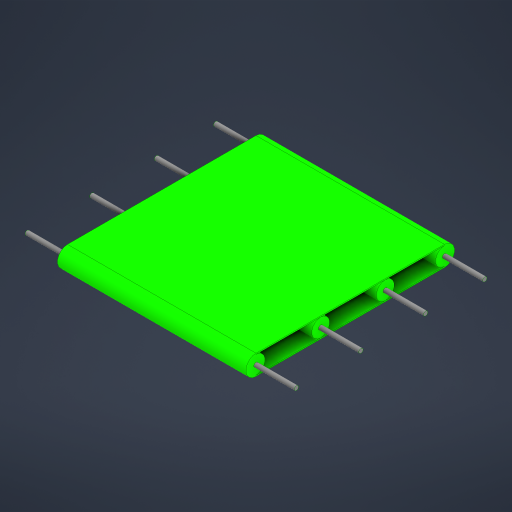
# Autodesk Inventor part: Conveyor
Saved by Autodesk Inventor 2023 (Build 270158000, 158)
## iProperties
Created: 2023-11-04
Part Number: Conveyor
Material: Generic
Document SubType Name: Modeling
Designer: Abhinav
Density: 1 g/cm^3
Appearance: Default(1)
Author: Abhinav
Autodesk Inventor part; units mm, degrees
ref_plane "YZ Plane" through (0, 0, 0) normal (1, 0, 0) x (0, 1, 0)
ref_plane "XZ Plane" through (0, 0, 0) normal (0, 1, 0) x (-1, 0, 0)
sketch "Sketch1" plane through (0, 0, 0) normal (1, 0, 0) x (0, 1, 0)
  line L0 (0, 0) -> (0, -350) construction
  line L1 (0, 0) -> (0, -350) construction
  line L2 (-16.7, 0) -> (-16.7, -350)
  line L3 (16.7, -350) -> (16.7, 0)
  arc A0 (16.7, 0) -> (-16.7, 0) centre (0, 0) ccw
  arc A1 (-16.7, -350) -> (16.7, -350) centre (0, -350) ccw
  line L4 (0, 0) -> (0, -350) construction
  line L5 (-18.7, 0) -> (-18.7, -350)
  line L6 (18.7, -350) -> (18.7, 0)
  arc A2 (18.7, 0) -> (-18.7, 0) centre (0, 0) ccw
  arc A3 (-18.7, -350) -> (18.7, -350) centre (0, -350) ccw
  circle A4 centre (0, 0) radius 16.7
  circle A5 centre (0, -350) radius 16.7
  line L7 (0, 0) -> (0, -120) construction
  line L8 (0, -120) -> (0, -240) construction
  circle A6 centre (0, -120) radius 16.7
  circle A7 centre (0, -240) radius 16.7
  point P0 (0, -175)
  point P1 (0, -175)
  point P2 (-16.7, -240)
  point P3 (-16.7, -120)
  point P4 (16.7, 0)
  point P5 (16.7, -120)
  point P6 (16.7, -240)
  point P7 (16.7, -350)
  dimension "d0" = 350
  dimension "d1" = 33.4
  dimension "d8" = 37.4
  dimension "d9" = 120
  dimension "d10" = 120
  constraints: 22 end point, 10 tangent, 8 point on circle, 6 centre point, 4 coincident, 3 equal length, 2 midpoint, 2 point on line, 2 vertical, 6 other
  measures "d0" distance of L0.start L0.end
  measures "d1" diameter of A1
  measures "d8" diameter of A3
  measures "d9" distance of L7.start L7.end
  measures "d10" distance of L7.end L8.end
extrude "Extrusion1" add sketch "Sketch1" along normal blind 350 contours A0 A4 | A6 | A7 | A5 A1 | A2 L6 A3 L5
sketch "Sketch2" plane through (350, 0, 0) normal (1, 0, 0) x (0, 0, -1)
  arc A0 (350, -16.7) -> (350, 25) centre (350, 0) ccw projected
  circle A1 centre (350, 0) radius 4
  circle A2 centre (240, 0) radius 4
  arc A3 (120, -16.7) -> (120, 16.7) centre (120, 0) ccw projected
  circle A4 centre (120, 0) radius 4
  arc A5 (0, -16.7) -> (0, 16.7) centre (0, 0) ccw projected
  circle A6 centre (0, 0) radius 4
  dimension "d7" = 8
  constraints: 4 centre point, 3 coincident, 3 equal radius, 1 other
  measures "d7" diameter of A1
extrude "Extrusion2" add sketch "Sketch2" along normal blind 75
ref_plane "Work Plane1" through (175, 0, 0) normal (-1, 0, 0) x (0, 0, 1)
mirror "Mirror1" about plane through (175, 0, 0) normal (-1, 0, 0) of "Extrusion2"
body "Solid1"
